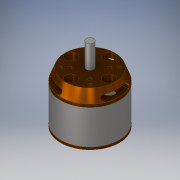
# Autodesk Inventor part: KEDA_6364
Saved by Autodesk Inventor 2019.2 (Build 232265000, 265)
## iProperties
Created: 2018-06-19
Part Number: KEDA_6364
Material: Generic
Document SubType Name: Modeling
Designer: Johansson
Density: 1 g/cm^3
Appearance: Default
Author: Johansson
Autodesk Inventor part; units mm, degrees
ref_plane "XZ Plane" through (0, 0, 0) normal (0, 1, 0) x (-1, 0, 0)
ref_plane "XY Plane" through (0, 0, 0) normal (0, 0, 1) x (1, 0, 0)
sketch "Sketch1" plane through (0, 0, 0) normal (0, 1, 0) x (-1, 0, 0)
  circle A0 centre (0, 0) radius 31.5
  dimension "d0" = 63
  constraints: 1 centre point, 1 coincident
  measures "d0" diameter of A0
extrude "Extrusion1" add sketch "Sketch1" along normal blind 37
sketch "Sketch2" plane through (0, 37, 0) normal (0, 1, 0) x (1, 0, 0)
  circle A0 centre (0, 0) radius 31.5
  constraints: 1 centre point, 1 coincident
extrude "Extrusion2" add sketch "Sketch2" along normal blind 15 separate body
chamfer "Chamfer1" distance 4.5 distance2 12 1 edges at (-31.5, 52, 0) measured on face at (8.757, 52, -9.3296)
sketch "Sketch3" plane through (0, 52, 0) normal (0, 1, 0) x (1, 0, 0)
  circle A0 centre (-20.5, 0) radius 6
  line L0 (-44.1, 0) -> (44.1, 0) projected
  line L1 (0, -33.1999) -> (0, 39.3545) construction
  circle A1 centre (20.5, 0) radius 6
  line L2 (0, 53.8654) -> (0, -47.7108) projected
  point P0 (0, 0)
  dimension "d8" = 12
  dimension "d9" = 41
  constraints: 2 centre point, 2 end point, 1 collinear, 1 point on line, 1 symmetric about line, 1 vertical, 1 other
  measures "d8" diameter of A0
  measures "d9" distance of A1.centre A0.centre
extrude "Extrusion3" cut sketch "Sketch3" against normal through all bodies 2
pattern_circular "Circular Pattern1" count 2 over 90 about axis through (0, -10, 0) along (0, 1, 0) of "Extrusion3" bodies 2
sketch "Sketch4" plane through (0, 52, 0) normal (0, 1, 0) x (1, 0, 0)
  line L0 (0, 0) -> (-16.213, 16.213) construction
  line L1 (0, 0) -> (22.9287, 0) construction
  line L2 (0, 0) -> (-7.0412, -7.0412) construction
  circle A0 centre (-16.0867, 16.0867) radius 2
  circle A1 centre (-10.7834, 10.7834) radius 2
  line L3 (0, 0) -> (16.213, -16.213) construction
  circle A2 centre (16.0867, -16.0867) radius 2
  circle A3 centre (10.7834, -10.7834) radius 2
  dimension "d15" = 135
  dimension "d16" = 4
  dimension "d17" = 4
  dimension "d18" = 3.5
  dimension "d19" = 26.5
  constraints: 8 end point, 4 centre point, 4 point on line, 3 symmetric about line, 1 equal length, 1 horizontal, 2 other
  measures "d15" angle of L1 L0
  measures "d16" diameter of A0
  measures "d17" diameter of A1
extrude "Extrusion4" cut sketch "Sketch4" against normal through all bodies 2
thread "Thread1" size "M4x0.7" class "6H" standard "ANSI Metric M Profile" full length
thread "Thread2" size "M4x0.7" class "6H" standard "ANSI Metric M Profile" full length
thread "Thread3" size "M4x0.7" class "6H" standard "ANSI Metric M Profile" full length
thread "Thread4" size "M4x0.7" class "6H" standard "ANSI Metric M Profile" full length
pattern_circular "Circular Pattern2" count 2 over 90 about axis through (0, -10, 0) along (0, 1, 0) of "Extrusion4" bodies 2
ref_plane "Work Plane1" through (31.5, 0, 0) normal (1, 0, 0) x (0, 1, 0)
sketch "Sketch5" plane through (31.5, 0, 0) normal (1, 0, 0) x (0, 1, 0)
  line L0 (43.2, -12) -> (43.2, 12) construction
  line L1 (46.2, -12) -> (46.2, 12)
  line L2 (40.2, 12) -> (40.2, -12)
  arc A0 (40.2, -12) -> (46.2, -12) centre (43.2, -12) ccw
  arc A1 (46.2, 12) -> (40.2, 12) centre (43.2, 12) ccw
  line L3 (52, 27) -> (52, -27) projected
  line L4 (-10.4, 0) -> (62.4, 0) projected
  point P0 (0, 0)
  point P1 (43.2, 0)
  dimension "d33" = 30
  dimension "d34" = 6
  dimension "d35" = 5.8
  constraints: 8 end point, 4 point on circle, 4 tangent, 2 centre point, 1 midpoint, 1 parallel, 1 point on line, 1 vertical
  measures "d34" distance between parallel lines of L2 L1
  measures "d35" distance between parallel lines of L3 L1
extrude "Extrusion5" cut sketch "Sketch5" against normal blind 10 bodies 2
pattern_circular "Circular Pattern3" count 3 over 360 about axis through (0, -10, 0) along (0, 1, 0) of "Extrusion5" bodies 2
sketch "Sketch6" plane through (0, 52, 0) normal (0, 1, 0) x (1, 0, 0)
  circle A0 centre (0, 0) radius 4
  dimension "d41" = 8
  constraints: 1 centre point, 1 coincident
  measures "d41" diameter of A0
extrude "Extrusion6" add sketch "Sketch6" along normal blind 25 separate body
sketch "Sketch7" plane through (0, 0, 0) normal (0, -1, 0) x (1, 0, 0)
  circle A0 centre (0, 0) radius 31.5 projected
extrude "Extrusion7" add sketch "Sketch7" along normal blind 15 separate body
chamfer "Chamfer2" distance 25.75 distance2 12.5 1 edges at (-31.5, -15, 0) measured on face at (8.757, -15, 9.3296)
